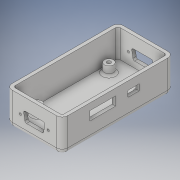
# Autodesk Inventor part: Motor_Node_box
Saved by Autodesk Inventor 2019 (Build 230136000, 136)
## iProperties
Created: 2019-12-12
Part Number: Motor_Node_box
Material: Generic
Document SubType Name: Modeling
Designer: Jorian Brusind
Density: 1 g/cm^3
Appearance: Default
Author: Jorian Brusind
Autodesk Inventor part; units mm, degrees
ref_plane "YZ Plane" through (0, 0, 0) normal (1, 0, 0) x (0, 1, 0)
ref_plane "XZ Plane" through (0, 0, 0) normal (0, 1, 0) x (-1, 0, 0)
sketch "Sketch1" plane through (0, 0, 0) normal (0, 1, 0) x (-1, 0, 0)
  line L0 (0, 0) -> (50, 0)
  line L1 (50, 0) -> (50, -100)
  line L2 (50, -100) -> (0, -100)
  line L3 (0, -100) -> (0, 0)
  dimension "d0" = 50
  dimension "d1" = 100
  constraints: 8 end point, 2 parallel, 1 horizontal, 1 perpendicular
  measures "d0" distance of L1.end L2.end
  measures "d1" distance of L0.end L1.end
extrude "Extrusion1" add sketch "Sketch1" along normal blind 30
sketch "Sketch2" plane through (0, 30, 0) normal (0, 1, 0) x (1, 0, 0)
  line L0 (-50, 0) -> (0, 0) projected
  line L1 (0, 0) -> (-3, 0)
  line L2 (-3, 0) -> (-3, 3)
  line L3 (-3, 3) -> (-47, 3)
  line L4 (-47, 3) -> (-47, 97)
  line L5 (-47, 97) -> (-3, 97)
  line L6 (-3, 97) -> (-3, 3)
  dimension "d4" = 3
  dimension "d5" = 3
  dimension "d6" = 44
  dimension "d7" = 94
  constraints: 12 end point, 2 parallel, 2 perpendicular, 1 horizontal, 1 point on line
  measures "d4" distance of L0.end L1.end
  measures "d5" distance of L1.end L2.end
  measures "d6" distance of L4.end L5.end
  measures "d7" distance of L3.end L4.end
extrude "Extrusion2" cut sketch "Sketch2" against normal blind 25
sketch "Sketch3" plane through (0, 5, 0) normal (0, 1, 0) x (1, 0, 0)
  line L0 (-3, 3) -> (-47, 3) projected
  line L1 (-25, 3) -> (-25, 34.3333)
  line L2 (-47, 97) -> (-3, 97) projected
  line L3 (-25, 97) -> (-25, 65.6667)
  circle A0 centre (-25, 34.3333) radius 2.75
  circle A1 centre (-25, 65.6667) radius 2.75
  point P0 (0, 0)
  dimension "d10" = 31.3333
  dimension "d11" = 31.3333
  dimension "d12" = 5.5
  dimension "d13" = 5.5
  constraints: 4 end point, 2 centre point, 2 coincident, 2 midpoint, 2 vertical
  measures "d10" distance of L1.start L1.end
  measures "d11" distance of L3.start L3.end
  measures "d12" diameter of A0
  measures "d13" diameter of A1
extrude "Extrusion3" cut sketch "Sketch3" against normal blind 15
sketch "Sketch4" plane through (0, 5, 0) normal (0, 1, 0) x (1, 0, 0)
  circle A0 centre (-40, 18) radius 4
  line L0 (-3, 3) -> (-47, 3) projected
  line L1 (-47, 3) -> (-47, 97) projected
  circle A1 centre (-40, 82) radius 4
  circle A2 centre (-10, 18) radius 4
  circle A3 centre (-10, 82) radius 4
  circle A4 centre (-40, 82) radius 1.75
  circle A5 centre (-40, 18) radius 1.75
  circle A6 centre (-10, 82) radius 1.75
  circle A7 centre (-10, 18) radius 1.75
  point P0 (0, 0)
  dimension "d16" = 8
  dimension "d17" = 15
  dimension "d18" = 7
  dimension "d21" = 64
  dimension "d24" = 30
  dimension "d27" = 3.5
  dimension "d30" = 64
  dimension "d33" = 30
  constraints: 8 centre point, 2 horizontal, 2 vertical, 1 coincident, 12 other
  measures "d16" diameter of A0
  measures "d17" distance from line of L0 A0.centre
  measures "d18" distance from line of L1 A0.centre
  measures "d21" distance of A0.centre A1.centre
  measures "d24" distance of A0.centre A2.centre
  measures "d27" diameter of A4
  measures "d30" distance of A4.centre A5.centre
  measures "d33" distance of A4.centre A6.centre
extrude "Extrusion4" add sketch "Sketch4" along normal blind 8
sketch "Sketch6" plane through (-50, 0, 0) normal (0, 0, 1) x (1, 0, 0)
  line L0 (50, 0) -> (50, 15)
  line L1 (50, 0) -> (50, 30) projected
  line L2 (50, 15) -> (25, 15)
  line L3 (25, 15) -> (12.5, 15)
  line L4 (25, 15) -> (37.5, 15)
  circle A0 centre (12.5, 15) radius 1
  circle A1 centre (37.5, 15) radius 1
  line L5 (25, 15) -> (25, 19.5)
  line L6 (25, 19.5) -> (17, 19.5)
  line L7 (25, 19.5) -> (33, 19.5)
  line L8 (25, 15) -> (25, 10.5)
  line L9 (25, 10.5) -> (32, 10.5)
  line L10 (25, 10.5) -> (18, 10.5)
  line L11 (17, 19.5) -> (17, 18)
  arc A2 (17, 19.5) -> (15.5, 18) centre (17, 18) ccw
  line L12 (18, 10.5) -> (18, 12)
  arc A3 (16.5, 12) -> (18, 10.5) centre (18, 12) ccw
  line L13 (16.5, 12) -> (15.5, 18)
  line L14 (32, 10.5) -> (32, 12)
  line L15 (33, 19.5) -> (33, 18)
  arc A4 (34.5, 18) -> (33, 19.5) centre (33, 18) ccw
  line L16 (33, 18) -> (34.5, 18) construction
  line L17 (33, 18) -> (33, 19.5) construction
  arc A5 (32, 10.5) -> (33.5, 12) centre (32, 12) ccw
  line L18 (34.5, 18) -> (33.5, 12)
  dimension "d48" = 25
  dimension "d49" = 12.5
  dimension "d50" = 12.5
  dimension "d51" = 2
  dimension "d52" = 2
  dimension "d53" = 4.5
  dimension "d54" = 8
  dimension "d55" = 8
  dimension "d56" = 4.5
  dimension "d57" = 7
  dimension "d58" = 7
  dimension "d59" = 1.5
  dimension "d60" = 1.5
  dimension "d61" = 1.5
  dimension "d62" = 90
  dimension "d63" = 1.5
  dimension "d64" = 90
  constraints: 36 end point, 8 point on circle, 6 centre point, 6 coincident, 4 horizontal, 4 vertical, 3 perpendicular, 2 midpoint
  measures "d48" distance of L0.end L2.end
  measures "d49" distance of L2.end L3.end
  measures "d50" distance of L2.end L4.end
  measures "d51" diameter of A0
  measures "d52" diameter of A1
  measures "d53" distance of L2.end L5.end
  measures "d54" distance of L5.end L6.end
  measures "d55" distance of L5.end L7.end
  measures "d56" distance of L2.end L8.end
  measures "d57" distance of L8.end L9.end
  measures "d58" distance of L8.end L10.end
  measures "d59" distance of L6.end L11.end
  measures "d60" distance of L10.end L12.end
  measures "d61" distance of L9.end L14.end
  measures "d62" angle of L9 L14
  measures "d63" distance of L7.end L15.end
  measures "d64" angle of L16 L17
extrude "Extrusion6" cut sketch "Sketch6" against normal blind 3
ref_plane "Work Plane1" through (0, 0, -50) normal (0, 0, 1) x (1, 0, 0)
mirror "Mirror1" about plane through (0, 0, -50) normal (0, 0, 1) of "Extrusion6"
sketch "Sketch7" plane through (0, 0, 0) normal (1, 0, 0) x (0, 0, -1)
  line L0 (24, 20) -> (49, 20)
  line L1 (100, 0) -> (100, 30) projected
  line L2 (49, 20) -> (36.5, 20)
  line L3 (49, 20) -> (64, 20)
  line L4 (25, 16) -> (48, 16)
  line L5 (48, 16) -> (48, 24)
  line L6 (48, 24) -> (25, 24)
  line L7 (25, 24) -> (25, 16)
  line L8 (25, 16) -> (48, 24) construction
  line L9 (48, 16) -> (25, 24) construction
  line L10 (58.8, 22.75) -> (69.2, 22.75)
  line L11 (69.2, 22.75) -> (69.2, 17.25)
  line L12 (69.2, 17.25) -> (58.8, 17.25)
  line L13 (58.8, 17.25) -> (58.8, 22.75)
  line L14 (58.8, 22.75) -> (69.2, 17.25) construction
  line L15 (69.2, 22.75) -> (58.8, 17.25) construction
  line L16 (100, 0) -> (0, 0) projected
  line L17 (0, 0) -> (0, 30) projected
  dimension "d68" = 25
  dimension "d69" = 15
  dimension "d70" = 23
  dimension "d71" = 8
  dimension "d72" = 10.4
  dimension "d73" = 5.5
  dimension "d76" = 20
  dimension "d77" = 25
  constraints: 30 end point, 5 midpoint, 4 parallel, 3 perpendicular, 2 horizontal, 1 point on line
  measures "d68" distance of L0.start L0.end
  measures "d69" distance of L0.end L3.end
  measures "d70" distance of L6.end L5.end
  measures "d71" distance of L5.end L4.end
  measures "d72" distance of L11.end L12.end
  measures "d73" distance of L10.end L11.end
  measures "d76" distance between parallel lines of L16 L0
  measures "d77" distance between parallel lines of L17 L7
extrude "Extrusion7" cut sketch "Sketch7" against normal blind 3
fillet "Fillet1" radius 5 4 edges at (0, 15, 0) (0, 15, -100) (-50, 15, -100) (-50, 15, 0)
fillet "Fillet2" radius 5 8 edges at (-1.4645, 0, -1.4645) (-25, 0, 0) (-48.5355, 0, -1.4645) (-50, 0, -50) (-48.5355, 0, -98.5355) (-25, 0, -100) (-1.4645, 0, -98.5355) (0, 0, -50)
fillet "Fillet3" radius 2 4 edges at (-44, 5, -18) (-44, 5, -82) (-14, 5, -18) (-14, 5, -82)
fillet "Fillet4" radius 2 4 edges at (-47, 17.5, -97) (-47, 17.5, -3) (-3, 17.5, -3) (-3, 17.5, -97)
fillet "Fillet5" radius 1 1 edges at (-1.5, 22.75, -58.8)
fillet "Fillet6" radius 1 1 edges at (-1.5, 17.25, -58.8)
body "Solid1"
